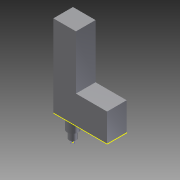
# Autodesk Inventor part: tool Part1
Saved by Autodesk Inventor 2012 (Build 160160000, 160)
## iProperties
Created: 2012-06-20
Part Number: tool Part1
Material: Default
Document SubType Name: Modeling
Designer: wberry
Density: 1 g/cm^3
Author: wberry
Autodesk Inventor part; units mm, degrees
ref_plane "YZ Plane" through (0, 0, 0) normal (1, 0, 0) x (0, 1, 0)
ref_plane "XZ Plane" through (0, 0, 0) normal (0, 1, 0) x (-1, 0, 0)
ref_plane "XY Plane" through (0, 0, 0) normal (0, 0, 1) x (1, 0, 0)
sketch "Sketch1" plane through (0, 0, 0) normal (0, 0, 1) x (1, 0, 0)
  line L0 (0, 0) -> (50.8, 0)
  line L1 (50.8, 63) -> (50.8, 184.15)
  line L2 (50.8, 184.15) -> (0, 184.15)
  line L3 (0, 184.15) -> (0, 0)
  line L4 (50.8, 0) -> (120.8, 0)
  line L5 (120.8, 0) -> (120.8, 63)
  line L6 (120.8, 63) -> (50.8, 63)
  line L7 (50.8, 63) -> (50.8, 0)
  dimension "d0" = 50.8
  dimension "d2" = 70
  dimension "d3" = 63
  constraints: 16 end point, 4 parallel, 2 horizontal, 2 perpendicular
  measures "d0" distance of L2.end L1.end
  measures "d2" distance of L1.start L5.end
  measures "d3" distance of L5.end L4.end
extrude "Extrusion2" add sketch "Sketch1" along normal blind 44.1
sketch "Sketch3" plane through (0, 0, 0) normal (0, -1, 0) x (1, 0, 0)
  line L0 (120.8, 44.1) -> (0, 44.1) projected
  line L1 (0, 0) -> (0, 44.1) projected
  line L2 (0, 0) -> (120.8, 0) projected
  line L3 (120.8, 0) -> (120.8, 44.1) projected
sketch "Sketch4" plane through (0, 0, 0) normal (0, -1, 0) x (1, 0, 0)
  circle A0 centre (21.61, 22.21) radius 12.5
  dimension "d8" = 25
  constraints: 1 centre point
  measures "d8" diameter of A0
extrude "Extrusion3" add sketch "Sketch4" along normal blind 32
sketch "Sketch5" plane through (21.61, -32, 22.21) normal (0, -1, 0) x (1, 0, 0)
  circle A0 centre (0, 0) radius 12.5 projected
  circle A1 centre (0, 0) radius 8
  point P0 (-21.61, -22.21)
  dimension "d12" = 16
  constraints: 1 centre point, 1 coincident
  measures "d12" diameter of A1
extrude "Extrusion4" add sketch "Sketch5" along normal blind 17.64 contours A1
sketch "Sketch6" plane through (21.61, -49.64, 22.21) normal (0, -1, 0) x (1, 0, 0)
  circle A0 centre (0, 0) radius 8 projected
  circle A1 centre (0, 0) radius 1.5
  point P0 (-21.61, -22.21)
  dimension "d15" = 3
  constraints: 1 centre point, 1 coincident
  measures "d15" diameter of A1
extrude "Extrusion5" add sketch "Sketch6" along normal blind 7 contours A1
sketch "Sketch7" plane through (21.61, -56.64, 22.21) normal (0, -1, 0) x (1, 0, 0)
  circle A0 centre (0, 0) radius 1.5 projected
  point P0 (-21.61, -22.21)
  constraints: 1 coincident
body "Solid2"
